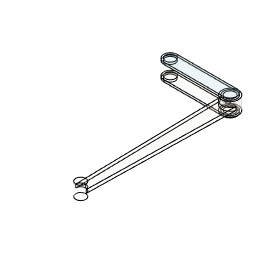
total chuck v28 (Autodesk Fusion 360 archive; units mm, degrees)
design "connection"
description: link the piston to the body
part number: connection
Autodesk Fusion 360 part; units mm, degrees
sketch "草图1" plane through (0, 0, 0) normal (0, 0, 1) x (1, 0, 0)
  circle A0 centre (0, 200) radius 0.75
  line L0 (0, 200) -> (9.007, 200)
  circle A1 centre (9.007, 200) radius 0.75
  dimension "d1" = 1.5
  dimension "d3" = 9.007
  dimension "d5" = 1.5
  constraint coincident A0.centre L0.start
  constraint horizontal L0
  constraint coincident L0.end A1.centre
  measures "d1" diameter of A0
  measures "d3" distance of A0.centre L0.end
  measures "d5" diameter of A1
extrude "拉伸1" add sketch "草图1" along normal mid plane 2 makes body 1 at (-0.64, 199.6089, 0.6667) makes body 2 at (8.2579, 199.9626, 0.3333)
sketch "草图2" plane through (0, 0, 1) normal (0, 0, 1) x (-1, 0, 0)
  circle A0 centre (0, -200) radius 0.75
  line L0 (-0.0328, -200.9995) -> (-9, -201)
  line L1 (-0.0328, -199.0005) -> (-9, -199)
  arc A1 (-0.0328, -200.9995) -> (-0.0328, -199.0005) centre (0, -200) ccw
  arc A2 (-9, -199) -> (-9, -201) centre (-9.0001, -200) ccw
  dimension "d8" = 2
  dimension "d9" = 2
  constraint concentric A0 A1
  constraint tangent L0 A2
  constraint tangent L1 A2
  measures "d8" diameter of A1
  measures "d9" diameter of A2
extrude "拉伸2" add sketch "草图2" along normal blind 0.3 bodies 2 1
mirror "镜像1" about plane through (0, 0, 0) normal (0, 0, 1) of "拉伸2"
copy_body "实体->零部件1" bodies 2 removing the originals makes body 3 in component "Component"
sketch "草图3" plane through (0, 0, 1.3) normal (0, 0, 1) x (-1, 0, 0)
  circle A0 centre (0, -200) radius 0.75
  arc A1 (-0.0328, -200.9995) -> (-0.0328, -199.0005) centre (0, -200) ccw
  line L0 (-0.0328, -199.0005) -> (-9, -199)
  arc A2 (-9, -199) -> (-9, -201) centre (-9.0001, -200) ccw
  line L1 (-9, -201) -> (-0.0328, -200.9995)
  dimension "d14" = 9.0001
  measures "d14" distance of A0.centre A2.centre
sketch "草图4" plane through (0, 0, 0) normal (0, 0, 1) x (1, 0, 0)
  line L0 (20, 200) -> (20.007, 200)
  line L1 (20.007, 200) -> (20.007, 177.5)
  circle A0 centre (20.007, 177.5) radius 0.75
  dimension "d17" = 0.007
  dimension "d18" = 22.5
  dimension "d19" = 1.5
  constraint horizontal L0
  constraint perpendicular L0 L1
  constraint coincident L1.end A0.centre
  measures "d17" distance of L0.start L0.end
  measures "d18" distance of L0.end L1.end
  measures "d19" diameter of A0
sketch "草图5" plane through (0, 0, 0) normal (0, 0, 1) x (1, 0, 0)
sketch "草图6" plane through (0, 0, 0) normal (0, 0, 1) x (1, 0, 0)
sketch "草图7" plane through (0, 0, 0) normal (0, 0, 1) x (1, 0, 0)
sketch "草图8" plane through (0, 0, 0) normal (0, 0, 1) x (1, 0, 0)
  circle A0 centre (20, 200) radius 1
  circle A1 centre (20, 200) radius 1.25
  dimension "d22" = 2
  dimension "d23" = 2.5
  constraint concentric A0 A1
  measures "d22" diameter of A0
  measures "d23" diameter of A1
extrude "拉伸3" add sketch "草图4" sketch "草图8" along normal mid plane 2 separate body of sketch 2 makes body 4 at (20.7345, 177.3178, 0.6667) makes body 5 at (21.1746, 199.5725, 0.6667)
sketch "草图9" plane through (0, 0, 0) normal (0, 0, 1) x (1, 0, 0)
  circle A0 centre (20, 200) radius 1.25
  circle A1 centre (20, 177.5) radius 0.75
  line L0 (18.7917, 199.68) -> (19.2502, 177.4845)
  line L1 (20.7498, 177.4845) -> (21.2083, 199.68)
  dimension "d26" = 2.5
  dimension "d27" = 1.5
  constraint coincident A0 L0.start
  constraint coincident A1 L0.end
  constraint tangent A1 L0
  constraint coincident A1 L1.start
  constraint coincident A0 L1.end
  constraint tangent A1 L1
  measures "d26" diameter of A0
  measures "d27" diameter of A1
extrude "拉伸4" add sketch "草图9" along normal mid plane 0.5 contours A0 A1 L0 L1 bodies 4 5
copy_body "实体->零部件2" bodies 4 removing the originals makes body 6 in component "Component'"
component "Component" placed x (1, 0, 0) y (0, 1, 0) z (0, 0, 1) at (0, 0, 0)
component "Component'" placed x (1, 0, 0) y (0, 1, 0) z (0, 0, 1) at (-10.993, 0, 0)
